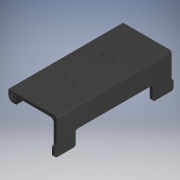
# Autodesk Inventor part: コックピット_サブフレーム_1_7_
Saved by Autodesk Inventor 2018 (Build 220112000, 112)
## iProperties
Created: 2018-06-13
Part Number: コックピット_サブフレーム_1_7_
Material: 一般
Document SubType Name: Modeling
Designer: taka
Density: 1 g/cm^3
Appearance: 滑らか - 黒
Author: taka
Autodesk Inventor part; units mm, degrees
ref_plane "YZ Plane" through (0, 0, 0) normal (1, 0, 0) x (0, 1, 0)
ref_plane "XZ Plane" through (0, 0, 0) normal (0, 1, 0) x (-1, 0, 0)
ref_plane "XY Plane" through (0, 0, 0) normal (0, 0, 1) x (1, 0, 0)
sketch "スケッチ1" plane through (0, 0, 0) normal (0, 1, 0) x (-1, 0, 0)
  line L0 (0, 0) -> (50, 0)
  line L1 (50, 0) -> (50, -118.5)
  line L2 (50, -118.5) -> (0, -118.5)
  line L3 (0, -118.5) -> (0, 0)
  dimension "d0" = 50
  dimension "d1" = 118.5
  constraints: 8 end point, 2 parallel, 1 horizontal, 1 perpendicular
  measures "d0" distance of L1.end L2.end
  measures "d1" distance of L0.end L1.end
extrude "押し出し1" add sketch "スケッチ1" along normal blind 3
sketch "スケッチ2" plane through (0, 0, 0) normal (0, -1, 0) x (1, 0, 0)
  line L0 (0, -118.5) -> (0, 0) projected
  line L1 (0, 0) -> (-3, 0)
  line L2 (-3, 0) -> (-3, -118.5)
  line L3 (-3, -118.5) -> (0, -118.5)
  line L4 (0, -118.5) -> (0, 0)
  line L5 (-50, -118.5) -> (0, -118.5) projected
  dimension "d4" = 3
  constraints: 8 end point, 2 collinear, 2 parallel, 1 horizontal, 1 perpendicular
  measures "d4" distance of L3.end L2.end
extrude "押し出し2" add sketch "スケッチ2" along normal blind 33
sketch "スケッチ3" plane through (0, 0, 0) normal (0, -1, 0) x (1, 0, 0)
  line L0 (-3, 0) -> (-50, 0) projected
  line L1 (-50, 0) -> (-50, -118.5) projected
  line L2 (-42, 0) -> (-50, 0)
  line L3 (-50, 0) -> (-50, -5)
  line L4 (-50, -5) -> (-42, -5)
  line L5 (-42, -5) -> (-42, 0)
  point P0 (0, 0)
  dimension "d7" = 8
  dimension "d8" = 5
  dimension "d9" = 8
  constraints: 8 end point, 2 parallel, 1 horizontal, 1 perpendicular, 1 point on line
  measures "d7" distance of L4.end L3.end
  measures "d8" distance between parallel lines of L0 L4
  measures "d9" distance between parallel lines of L5 L1
extrude "押し出し3" add sketch "スケッチ3" along normal blind 7
chamfer "面取り2" distance 7 angle 45 1 edges at (-42, 0, -2.5)
sketch "スケッチ4" plane through (-50, 3, 0) normal (0, 0, 1) x (1, 0, 0)
  line L0 (8, -3) -> (8, -10) projected
  line L1 (8, -10) -> (0, -10) projected
  line L2 (4.5, -5) -> (7.8, -5)
  line L3 (7.8, -5) -> (6.15, -7.8579)
  line L4 (6.15, -7.8579) -> (2.85, -7.8579)
  line L5 (2.85, -7.8579) -> (1.2, -5)
  line L6 (1.2, -5) -> (2.85, -2.1421)
  line L7 (2.85, -2.1421) -> (6.15, -2.1421)
  line L8 (6.15, -2.1421) -> (7.8, -5)
  line L9 (0, 0) -> (50, 0) projected
  point P0 (50, -3)
  dimension "d13" = 3.5
  dimension "d20" = 3.3
  dimension "d96" = 5
  constraints: 14 end point, 1 coincident, 1 horizontal, 13 other
  measures "d13" distance from line of L0 L2.start
  measures "d20" distance of L2.start L2.end
  measures "d96" distance from line of point (4.5, -5) L9
extrude "押し出し4" cut sketch "スケッチ4" against normal blind 2.5
fillet "フィレット1" radius 5 1 edges at (-50, -7, -2.5)
sketch "スケッチ6" plane through (-50, 3, 0) normal (0, 0, 1) x (1, 0, 0)
  line L0 (7.8, -5) -> (6.15, -7.8579) projected
  line L1 (6.15, -2.1421) -> (7.8, -5) projected
  line L2 (2.85, -2.1421) -> (6.15, -2.1421) projected
  line L3 (1.2, -5) -> (2.85, -2.1421) projected
  line L4 (2.85, -7.8579) -> (1.2, -5) projected
  line L5 (6.15, -7.8579) -> (2.85, -7.8579) projected
  circle A0 centre (4.5, -5) radius 1.65
  point P0 (50, -3)
  dimension "d24" = 3.3
  dimension "d25" = 6.6
  dimension "d26" = 3.3
  dimension "d27" = 5.7158
  dimension "d28" = 2.8579
  constraints: 1 centre point
  measures "d24" diameter of A0
  measures "d25" distance of L3.start L0.start
  measures "d26" distance of A0.centre L0.start
  measures "d27" distance between parallel lines of L2 L5
  measures "d28" distance from line of L5 A0.centre
extrude "押し出し5" cut sketch "スケッチ6" against normal through all contours A0
sketch "スケッチ7" plane through (-35, 0, -5) normal (0, 0, -1) x (-1, 0, 0)
  circle A0 centre (10.5, -2) radius 1.65 projected
  line L0 (0, 0) -> (15, 0) projected
  line L1 (10, -7) -> (7, -7) projected
  arc A1 (10, -7) -> (15, -2) centre (10, -2) ccw projected
  line L2 (15, 0) -> (15, -2) projected
  line L3 (7, -7) -> (0, 0) projected
  point P0 (-35, 0)
extrude "押し出し6" add sketch "スケッチ7" along normal blind 113.5
sketch "スケッチ8" plane through (0, 3, -118.5) normal (0, 0, -1) x (-1, 0, 0)
  circle A0 centre (45.5, -5) radius 1.65 projected
  line L0 (45.5, -5) -> (42.2, -5)
  line L1 (42.2, -5) -> (43.85, -2.1421)
  line L2 (43.85, -2.1421) -> (47.15, -2.1421)
  line L3 (47.15, -2.1421) -> (48.8, -5)
  line L4 (48.8, -5) -> (47.15, -7.8579)
  line L5 (47.15, -7.8579) -> (43.85, -7.8579)
  line L6 (43.85, -7.8579) -> (42.2, -5)
  point P0 (0, -3)
  dimension "d33" = 3.3
  constraints: 14 end point, 1 coincident, 1 horizontal, 13 other
  measures "d33" distance of L0.start L0.end
extrude "押し出し7" cut sketch "スケッチ8" against normal blind 2.4
sketch "スケッチ9" plane through (0, 0, 0) normal (0, -1, 0) x (1, 0, 0)
  line L0 (-35, 0) -> (-35, -118.5) projected
  line L1 (-3, 0) -> (-35, 0) projected
  line L2 (-35, -5) -> (-58.1779, -5)
  line L3 (-58.1779, -5) -> (-58.1779, -113.5)
  line L4 (-58.1779, -113.5) -> (-35, -113.5)
  line L5 (-35, -113.5) -> (-35, -5)
  point P0 (0, 0)
  point P1 (-42, 0)
  dimension "d36" = 5
  dimension "d37" = 108.5
  constraints: 8 end point, 2 parallel, 1 horizontal, 1 perpendicular, 1 point on line
  measures "d36" distance between parallel lines of L1 L2
  measures "d37" distance between parallel lines of L4 L2
extrude "押し出し8" cut sketch "スケッチ9" along normal through all
fillet "フィレット2" radius 4 1 edges at (-3, 0, -59.25)
fillet "フィレット3" radius 2 1 edges at (0, 3, -59.25)
sketch "スケッチ10" plane through (-3, -33, -118.5) normal (-1, 0, 0) x (0, 0, 1)
  line L0 (0, 29) -> (118.5, 29) projected
  line L1 (0, 29) -> (0, 0) projected
  line L2 (118.5, 0) -> (0, 0) projected
  line L3 (118.5, 29) -> (118.5, 0) projected
  line L4 (99.25, 0) -> (19.25, 0)
  line L5 (19.25, 0) -> (19.25, 15)
  line L6 (19.25, 15) -> (99.25, 15)
  line L7 (99.25, 15) -> (99.25, 0)
  point P0 (118.5, 33)
  dimension "d42" = 80
  dimension "d43" = 15
  dimension "d44" = 118.5
  dimension "d45" = 19.25
  constraints: 8 end point, 2 parallel, 1 horizontal, 1 perpendicular, 1 point on line
  measures "d42" distance of L5.end L6.end
  measures "d43" distance between parallel lines of L6 L2
  measures "d44" distance between parallel lines of L1 L3
  measures "d45" distance between parallel lines of L3 L7
extrude "押し出し9" cut sketch "スケッチ10" against normal through all contours L5 L6 L7 L2
sketch "スケッチ11" plane through (-3, -33, 0) normal (-1, 0, 0) x (0, 0, 1)
  line L0 (-99.25, 0) -> (-99.25, 15) projected
  line L1 (-99.25, 15) -> (-19.25, 15) projected
  line L2 (-19.25, 15) -> (-19.25, 0) projected
  line L3 (0, 0) -> (-19.25, 0) projected
  line L4 (0, 29) -> (0, 0) projected
  line L5 (-118.5, 29) -> (0, 29) projected
  line L6 (-118.5, 29) -> (-118.5, 0) projected
  line L7 (-99.25, 0) -> (-118.5, 0) projected
  line L8 (-118.5, 10) -> (-113.5, 10)
  line L9 (-113.5, 10) -> (-113.5, 22)
  line L10 (-113.5, 22) -> (-118.5, 22)
  line L11 (-118.5, 22) -> (-118.5, 10)
  point P0 (0, 33)
  dimension "d48" = 5
  dimension "d49" = 12
  dimension "d50" = 10
  constraints: 8 end point, 2 parallel, 1 horizontal, 1 perpendicular, 1 point on line
  measures "d48" distance of L10.end L9.end
  measures "d49" distance of L9.end L8.end
  measures "d50" distance between parallel lines of L7 L8
extrude "押し出し10" add sketch "スケッチ11" along normal blind 10 contours L6 L10 L9 L8
sketch "スケッチ13" plane through (-3, -23, -113.5) normal (0, 0, 1) x (1, 0, 0)
  line L0 (3, -10) -> (3, 24) projected
  line L1 (0, 0) -> (-10, 0) projected
  line L2 (0, 12) -> (-10, 12) projected
  line L3 (-4, 6) -> (-4, 9.3)
  line L4 (-4, 9.3) -> (-1.1421, 7.65)
  line L5 (-1.1421, 7.65) -> (-1.1421, 4.35)
  line L6 (-1.1421, 4.35) -> (-4, 2.7)
  line L7 (-4, 2.7) -> (-6.8579, 4.35)
  line L8 (-6.8579, 4.35) -> (-6.8579, 7.65)
  line L9 (-6.8579, 7.65) -> (-4, 9.3)
  line L10 (0, 19) -> (0, -10) projected
  line L11 (-10, 0) -> (-10, 12) projected
  point P0 (3, 23)
  dimension "d56" = 7
  dimension "d57" = 12
  dimension "d58" = 6
  dimension "d59" = 3.3
  constraints: 14 end point, 1 coincident, 1 vertical, 13 other
  measures "d56" distance from line of L0 L3.start
  measures "d57" distance between parallel lines of L2 L1
  measures "d58" distance from line of L2 L3.start
  measures "d59" distance of L3.start L3.end
extrude "押し出し11" cut sketch "スケッチ13" against normal blind 2.4 contours L4 L5 L6 L7 L8 L9
sketch "スケッチ14" plane through (0, -33, -118.5) normal (0, 0, -1) x (-1, 0, 0)
  line L0 (3, 0) -> (0, 0) projected
  line L1 (13, 22) -> (13, 10) projected
  line L2 (0, 34) -> (0, 0) projected
  circle A0 centre (7, 16) radius 1.75
  line L3 (3, 10) -> (13, 10) projected
  line L4 (3, 22) -> (13, 22) projected
  point P0 (0, 33)
  dimension "d62" = 3.5
  dimension "d63" = 6
  dimension "d64" = 16
  dimension "d65" = 12
  dimension "d66" = 10
  constraints: 1 centre point
  measures "d62" diameter of A0
  measures "d63" distance from line of L1 A0.centre
  measures "d64" distance from line of A0.centre L0
  measures "d65" distance between parallel lines of L3 L4
  measures "d66" distance between parallel lines of L0 L3
extrude "押し出し12" cut sketch "スケッチ14" against normal through all
fillet "フィレット4" radius 2 5 edges at (-8, -23, -113.5) (-8, -11, -113.5) (-13, -17, -113.5) (-13, -11, -116) (-13, -23, -116)
sketch "スケッチ15" plane through (0, -33, -118.5) normal (0, 0, -1) x (-1, 0, 0)
  line L0 (3, 0) -> (0, 0) projected
  line L1 (3, 10) -> (11, 10) projected
  line L2 (0, 34) -> (0, 0) projected
  line L3 (3, 10) -> (0, 10)
  line L4 (0, 10) -> (0, 0)
  line L5 (0, 0) -> (3, 0)
  line L6 (3, 0) -> (3, 10)
  point P0 (0, 33)
  constraints: 8 end point, 2 parallel, 1 horizontal, 1 perpendicular
extrude "押し出し13" add sketch "スケッチ15" along normal blind 2
sketch "スケッチ16" plane through (-3, -33, 0) normal (0, 0, 1) x (1, 0, 0)
  arc A0 (3, 34) -> (1, 36) centre (1, 34) ccw projected
  line L0 (-47, 36) -> (1, 36) projected
  line L1 (-39, 26) -> (-42, 26) projected
  line L2 (-4, 33) -> (-32, 33) projected
  arc A1 (0, 29) -> (-4, 33) centre (-4, 29) ccw projected
  line L3 (0, 29) -> (0, 0) projected
  line L4 (3, 0) -> (0, 0) projected
  line L5 (3, 0) -> (3, 34) projected
  line L6 (-40.85, 33.8579) -> (-39.2, 31) projected
  line L7 (-39.2, 31) -> (-40.85, 28.1421) projected
  line L8 (-40.85, 28.1421) -> (-44.15, 28.1421) projected
  line L9 (-44.15, 28.1421) -> (-45.8, 31) projected
  line L10 (-45.8, 31) -> (-44.15, 33.8579) projected
  line L11 (-44.15, 33.8579) -> (-40.85, 33.8579) projected
  line L12 (-8, 10) -> (0, 10) projected
  line L13 (3, 0) -> (0, 0)
  line L14 (0, 0) -> (0, 10)
  line L15 (0, 10) -> (3, 10)
  line L16 (3, 10) -> (3, 0)
  arc A2 (-47, 31) -> (-42, 26) centre (-42, 31) ccw projected
  line L17 (-47, 36) -> (-47, 31) projected
  line L18 (-32, 33) -> (-39, 26) projected
  point P0 (3, 33)
  constraints: 8 end point, 2 parallel, 1 horizontal, 1 perpendicular
extrude "押し出し14" add sketch "スケッチ16" along normal blind 2 contours L5 L4 L3 L15
sketch "スケッチ17" plane through (-50, 0, -113.5) normal (0, 0, 1) x (1, 0, 0)
  circle A0 centre (4.5, -2) radius 1.65 projected
  circle A1 centre (4.5, -2) radius 3
  point P0 (50, 0)
  dimension "d76" = 6
  constraints: 1 centre point, 1 coincident
  measures "d76" diameter of A1
extrude "押し出し15" cut sketch "スケッチ17" along normal blind 8
sketch "スケッチ18" plane through (-35, 0, -5) normal (0, 0, -1) x (-1, 0, 0)
  circle A0 centre (10.5, -2) radius 1.65 projected
  circle A1 centre (10.5, -2) radius 3
  point P0 (-35, 0)
  dimension "d79" = 6
  constraints: 1 centre point, 1 coincident
  measures "d79" diameter of A1
extrude "押し出し16" cut sketch "スケッチ18" along normal blind 8
fillet "フィレット6" radius 2 9 edges at (-1.5, -23, 2) (-1.5, -33, 2) (-1.5, -33, -19.25) (-1.5, -33, -99.25) (-1.5, -18, -99.25) (-1.5, -33, -120.5) (-1.5, -18, -19.25) (-1.5, -23, -120.5) (-50, 0, -59.25)
sketch "スケッチ19" plane through (0, 3, 0) normal (0, 1, 0) x (1, 0, 0)
  line L0 (-31.5, 79.25) -> (-21.5, 79.25)
  line L1 (-21.5, 79.25) -> (-21.5, 39.25)
  line L2 (-21.5, 39.25) -> (-31.5, 39.25)
  line L3 (-31.5, 39.25) -> (-31.5, 79.25)
  line L4 (-50, 118.5) -> (-50, 0) projected
  line L5 (-3, 97.25) -> (-3, 21.25) projected
  line L6 (-2, 118.5) -> (-50, 118.5) projected
  line L7 (-50, 0) -> (-2, 0) projected
  circle A0 centre (-31.5, 79.25) radius 0.9
  circle A1 centre (-21.5, 79.25) radius 0.9
  circle A2 centre (-31.5, 39.25) radius 0.9
  circle A3 centre (-21.5, 39.25) radius 0.9
  point P0 (0, 0)
  dimension "d83" = 10
  dimension "d84" = 40
  dimension "d85" = 47
  dimension "d86" = 118.5
  dimension "d87" = 39.25
  dimension "d88" = 18.5
  dimension "d89" = 1.8
  dimension "d90" = 1.8
  dimension "d91" = 1.8
  dimension "d92" = 1.8
  constraints: 8 end point, 4 centre point, 4 coincident, 2 parallel, 1 horizontal, 1 perpendicular
  measures "d83" distance of L1.end L2.end
  measures "d84" distance of L0.end L1.end
  measures "d85" distance between parallel lines of L5 L4
  measures "d86" distance between parallel lines of L7 L6
  measures "d87" distance between parallel lines of L6 L0
  measures "d88" distance between parallel lines of L4 L3
  measures "d89" diameter of A0
  measures "d90" diameter of A1
  measures "d91" diameter of A2
  measures "d92" diameter of A3
extrude "押し出し17" cut sketch "スケッチ19" against normal through all contours L3 A0 L0 | L0 A0 L3 | A1 L1 L0 | L0 L1 A1 | A2 L2 L3 | L3 L2 A2 | A3 L2 L1 | L1 L2 A3
equation "\"d9\" = d7"
equation "\"d26\" = 0.5 * d25"
equation "\"d28\" = 0.5 * d27"
equation "\"d45\" = -0.5 * d42 + 0.5 * d44"
equation "\"d58\" = 0.5 * d57"
equation "\"d64\" = 0.5 * d65 + d66"
equation "\"d87\" = -0.5 * d84 + 0.5 * d86"
equation "\"d88\" = -0.5 * d83 + 0.5 * d85"
equation "\"d90\" = d89"
equation "\"d91\" = d89"
equation "\"d92\" = d89"
